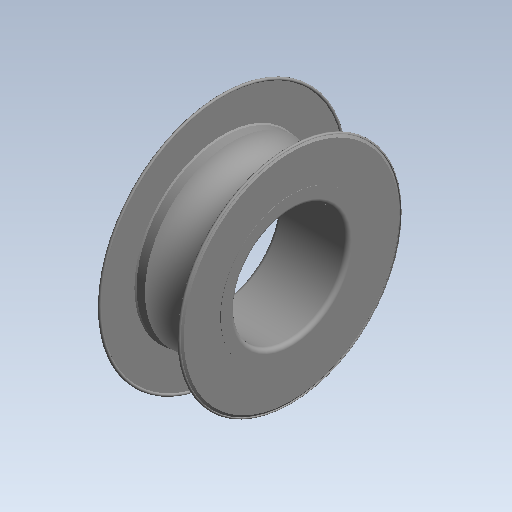
# Autodesk Inventor part: 7306 BE-2RZP_PART1
Saved by Autodesk Inventor 2020 (Build 240168000, 168)
## iProperties
Part Number: 7306 BE-2RZP_PART1
Material: Generic
Catalog Web Link: www.cadenas.de
Description: -Angular contact ball bearings, single row
Vendor: SKF
Document SubType Name: Modeling
Designer: partserver
Manufacturer: SKF
Mass: 12.4106 g
Surface Area: 126.875 cm^2
Volume: 12.4106 cm^3
Density: 1 g/cm^3
Appearance: PSOLRGB-175-175-175
Category: PARTsolutions
Company: SKF
PSOL_IDENT_0: {$CADENAS_DATA\23d-libs\skf\bearings_units_and_housings\ball_bearings\angular_contact_ball_bearings\
PSOL_IDENT_1: ba1_001_101.prj},204 {VTYP=3D},{NB=7306 BE-2RZP_PART1},{LINA=7306 BE-2RZP_PART1},{NN=BA1_001_101_PAR
PSOL_IDENT_2: T1},{NOPRJ=TRUE},{DATE=10.08.2020 12:45:11},{GEOMDATE=10.08.2020 08:19:26},{VERSION=},{LINEID=142100
PSOL_IDENT_3: },{WBVAR=},{WBNUMERIC=}  {NB=7306 BE-2RZP_PART1},{LINA=7306 BE-2RZP_PART1},{KT=DUMMY},{DESIGNATION=7
PSOL_IDENT_4: 306 BE-2RZP},{DD=30.000},{D=72.000},{B=19.0000},{DD1=46.500},{DD2=37.900},{D1=MIN},{D2=58.750},{D3=M
PSOL_IDENT_5: IN},{D4=64.260},{D5=64.85},{C1=MIN},{AA=31},{R12=1.100},{R34=0.600},{ALPHA=40},{PITCH=51.000},{DW=13
PSOL_IDENT_6: .494},{DDAMIN=37},{DDAMAX=46},{DAMAX=65},{DBMAX=67.8},{RAMAX=1},{RBMAX=0.6},{LOAD1=32.5},{LOAD2=19.3
PSOL_IDENT_7: },{LOAD3=0.815},{SPEED1=12000},{SPEED2=9500},{Z=10},{II=1},{MASS=0.35},{BEARING=7306 BE-2RZP},{POPUL
PSOL_IDENT_8: AR=Yes},{VARIANT=design_ba1_001_101_1},{D2A=58.75},{DD2A=37.900},{R5R=0.6},{R34L=1.1},{IRH=1},{ORH=1
PSOL_IDENT_9: },{D4H=1.1}
NB: 7306 BE-2RZP_PART1
NT: Angular contact ball bearings, single row
NBSYN: $DESIGNATION._PART1
LINA: 7306 BE-2RZP_PART1
CATALOG: SKF
SUPPLIER: SKF
ARTICLENO: 7306 BE-2RZP_PART1
BOMINFO: 7306 BE-2RZP_PART1
CREATOR: CADENAS GmbH
Title: 7306 BE-2RZP_PART1
Author: Cadenas PARTsolutions
Comments: Angular contact ball bearings, single row
Autodesk Inventor part; units mm, degrees
ref_plane "YZ Plane" through (0, 0, 0) normal (1, 0, 0) x (0, 1, 0)
ref_plane "XZ Plane" through (0, 0, 0) normal (0, 1, 0) x (-1, 0, 0)
ref_plane "XY Plane" through (0, 0, 0) normal (0, 0, 1) x (1, 0, 0)
sketch "Sketch_4" plane through (0, 0, 0) normal (0, 0, 1) x (1, 0, 0)
  line L0 (19, 0) -> (0, 0)
  line L1 (0, 18.95) -> (0, 16.1)
  arc A0 (0, 16.1) -> (1.1, 15) centre (1.1, 16.1) ccw
  line L2 (1.1, 15) -> (17.9, 15)
  arc A1 (17.9, 15) -> (19, 16.1) centre (17.9, 16.1) ccw
  line L3 (19, 16.1) -> (19, 23.25)
  line L4 (19, 23.25) -> (15.8608, 23.25)
  arc A2 (7.8815, 18.95) -> (15.8608, 23.25) centre (9.5, 25.5) ccw
  line L5 (7.8815, 18.95) -> (0, 18.95)
  constraints: 12 end point, 6 point on circle, 3 centre point
revolve "Revolution1" add sketch "Sketch_4" angle 360 about axis through (19, 0, 0) along (1, 0, 0)
sketch "Sketch_5" plane through (0, 0, 0) normal (0, 0, 1) x (1, 0, 0)
  line L0 (5, 0) -> (-5, 0)
  line L1 (0.0733, 28.7125) -> (0.0733, 18.95)
  line L2 (0.0733, 18.95) -> (0.9167, 18.95)
  line L3 (0.9167, 18.95) -> (0.6233, 19.2433)
  line L4 (0.6233, 19.2433) -> (0.6233, 29.0157)
  arc A0 (0.6233, 29.0157) -> (0.1833, 29.375) centre (0.55, 29.375) ccw
  line L5 (0.1833, 29.375) -> (0.3997, 29.375)
  arc A1 (0.4622, 29.253) -> (0.3997, 29.375) centre (0.3997, 29.298) ccw
  line L6 (0.4622, 29.253) -> (0.0733, 28.7125)
  constraints: 14 end point, 4 point on circle, 2 centre point
revolve "Revolution2" add sketch "Sketch_5" angle 360 about axis through (5, 0, 0) along (1, 0, 0)
sketch "Sketch_6" plane through (0, 0, 0) normal (0, 0, 1) x (1, 0, 0)
  line L0 (5, 0) -> (-5, 0)
  arc A0 (18.8167, 32.6875) -> (18.3767, 32.3282) centre (18.45, 32.6875) ccw
  line L1 (18.3767, 32.3282) -> (18.3767, 23.5433)
  line L2 (18.3767, 23.5433) -> (18.0833, 23.25)
  line L3 (18.0833, 23.25) -> (18.9267, 23.25)
  line L4 (18.9267, 23.25) -> (18.9267, 32.3875)
  line L5 (18.9267, 32.3875) -> (18.7082, 32.525)
  arc A1 (18.755, 32.6875) -> (18.7082, 32.525) centre (18.755, 32.5995) ccw
  line L6 (18.755, 32.6875) -> (18.8167, 32.6875)
  constraints: 14 end point, 4 point on circle, 2 centre point
revolve "Revolution3" add sketch "Sketch_6" angle 360 about axis through (5, 0, 0) along (1, 0, 0)
body "Solid1"
